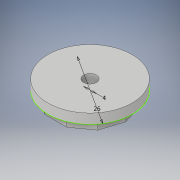
# Autodesk Inventor part: Probe P3
Saved by Autodesk Inventor 2019 (Build 230136000, 136)
## iProperties
Created: 2019-07-29
Part Number: Probe P3
Material: Generic
Document SubType Name: Modeling
Designer: azriel
Density: 1 g/cm^3
Appearance: Default
Author: azriel
Autodesk Inventor part; units mm, degrees
ref_plane "YZ Plane" through (0, 0, 0) normal (1, 0, 0) x (0, 1, 0)
ref_plane "XZ Plane" through (0, 0, 0) normal (0, 1, 0) x (-1, 0, 0)
ref_plane "XY Plane" through (0, 0, 0) normal (0, 0, 1) x (1, 0, 0)
sketch "Sketch1" plane through (0, 0, 0) normal (0, 1, 0) x (-1, 0, 0)
  circle A0 centre (0, 0) radius 13
  line L0 (-11.1, 0) -> (-8.9801, 6.5244)
  line L1 (-8.9801, 6.5244) -> (-3.4301, 10.5567)
  line L2 (-3.4301, 10.5567) -> (3.4301, 10.5567)
  line L3 (3.4301, 10.5567) -> (8.9801, 6.5244)
  line L4 (8.9801, 6.5244) -> (11.1, 0)
  line L5 (11.1, 0) -> (8.9801, -6.5244)
  line L6 (8.9801, -6.5244) -> (3.4301, -10.5567)
  line L7 (3.4301, -10.5567) -> (-3.4301, -10.5567)
  line L8 (-3.4301, -10.5567) -> (-8.9801, -6.5244)
  line L9 (-8.9801, -6.5244) -> (-11.1, 0)
  circle A1 centre (0, 0) radius 2
  dimension "d0" = 26
  dimension "d4" = 4
  constraints: 20 end point, 2 centre point, 2 coincident, 21 other
  measures "d0" diameter of A0
  measures "d4" diameter of A1
extrude "Extrusion2" add sketch "Sketch1" against normal blind 3 contours L0 L1 L2 L3 L4 L5 L6 L7 L8 L9
extrude "Extrusion3" add sketch "Sketch1" along normal blind 3 contours A0 | L0 L1 L2 L3 L4 L5 L6 L7 L8 L9
body "Solid2"
